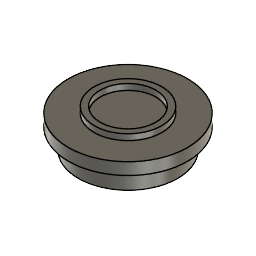
Boton Circulo (Autodesk Fusion 360 design; units mm, degrees)
Autodesk Fusion 360 part; units mm, degrees
sketch "Boceto1" plane through (0, 0, 0) normal (0, 0, 1) x (1, 0, 0)
  circle A0 centre (0, 0) radius 12.5
  dimension "d1" = 25
  constraint coincident A0.centre origin
  measures "d1" diameter of A0
extrude "Extruir1" add sketch "Boceto1" along normal blind 5
sketch "Boceto2" plane through (0, 0, 5) normal (0, 0, 1) x (-1, 0, 0)
  circle A0 centre (0, 0) radius 12.5
  circle A1 centre (0, 0) radius 15
  dimension "d4" = 30
  constraint concentric A0 A1
  measures "d4" diameter of A1
extrude "Extruir2" add sketch "Boceto2" along normal blind 3 contours A0 | A1
shell "Vaciado1" thickness 1.5 removed faces 1 at (-3.3879, -0.621, 0)
sketch "Boceto4" plane through (0, 0, 8) normal (0, 0, 1) x (-1, 0, 0)
  circle A0 centre (0, 0) radius 15
  circle A1 centre (0, 0) radius 8.5
  circle A2 centre (0, 0) radius 7
  dimension "d8" = 17
  dimension "d13" = 14
  constraint coincident A0.centre A1.centre
  constraint concentric A0 A2
  measures "d8" diameter of A1
  measures "d13" diameter of A2
extrude "Extruir3" add sketch "Boceto4" along normal blind 1.5 contours A1
